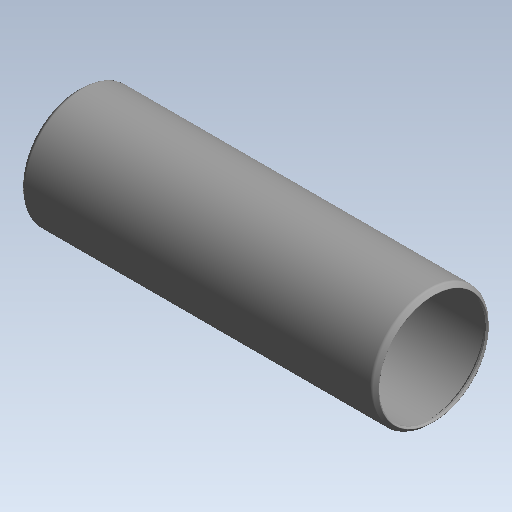
# Autodesk Inventor part: 09R-3.31350SR
Saved by Autodesk Inventor 2020 (Build 240168000, 168)
## iProperties
Part Number: 09R-3.31350SR
Material: Generic
Catalog Web Link: www.cadenas.de
Description: Tube-Original Line - Standard Air Cylinders
Vendor: BIMBA
Document SubType Name: Modeling
Designer: partserver
Manufacturer: BIMBA
Mass: 3.98472 g
Surface Area: 150.377 cm^2
Volume: 3.98472 cm^3
Density: 1 g/cm^3
Appearance: PSOLRGB-180-180-180
Category: PARTsolutions
Company: BIMBA
PSOL_IDENT_0: {$CADENAS_DATA\23d-libs\bimba\bimba_brand\bimba_imperial\bimba_full_line\original_line_cylinders\sta
PSOL_IDENT_1: ndard_air_cylinders\tube.prj},205 {VTYP=3D},{NB=09R-3.31350SR},{LINA=09R-3.31350SR},{NN=Tube},{DATE=
PSOL_IDENT_2: 19.01.2022 10:19:38},{GEOMDATE=03.03.2020 12:52:40},{VERSION=},{LINEID=60},{WBVAR=MNT,ACTING,NR,L,FO
PSOL_IDENT_3: URHOLES,SR,K},{WBNUMERIC=L,FOURHOLES}  {NB=09R-3.31350SR},{LINA=09R-3.31350SR},{KT=DUMMY},{PN=09R-3.
PSOL_IDENT_4: 31350SR},{BORE=1.06250000},{BOREPN=09},{MNT=},{MNTALG='' , 'Front Nose' , 'BF' , 'Front Block' , 'BF
PSOL_IDENT_5: T' , 'Front Trunnion' , 'A' , 'Adjustable Stroke'},{ACTING=R},{ACTINGALG= '' , 'Single Acting' , 'R'
PSOL_IDENT_6: , 'Reverse/Double Acting' },{NR=},{NRALG= '' , 'N/A' },{L=3.3135},{OD=1.1130},{ODN=1.1130},{ODP=1.1
PSOL_IDENT_7: 130},{ODB=1.1410},{ID=1.0715},{DV=0.00000000},{LV=0.00000000},{LV1=0.00000000},{G=0.0300},{FOURHOLES=
PSOL_IDENT_8: 0},{AA=0.3750},{BB=0.0940},{SR=SR},{SRALG= 'C' , 'Carbon Steel Rod' , 'SR' , '303 Stainless Steel Ro
PSOL_IDENT_9: d' , '' , '303 Stainless Steel Rod'},{KALG= '', 'Standard' , 'K' , 'Ports Rotated 90deg' },{K=}
NB: 09R-3.31350SR
NN: Tube
NT: Original Line - Standard Air Cylinders
NBSYN: $PN.
LINA: 09R-3.31350SR
CATALOG: Bimba Products
BORE: 0
BOREPN: 09
MNT: Front Nose
MNTALG: '' , 'Front Nose' , 'BF' , 'Front Block' , 'BFT' , 'Front Trunnion' , 'A' , 'Adjustable Stroke'
ACTING: Reverse/Double Acting
NR: N/A
L: 3.3135
ODN: 1.113
ODP: 1.113
ODB: 1.141
ID: 1.0715
DV: 0
LV: 0
LV1: 0
G: 0.03
FOURHOLES: 0
AA: 0.375
BB: 0.094
SR: 303 Stainless Steel Rod
K: Standard
SUPPLIER: BIMBA
ARTICLENO: 09R-3.31350SR
BOMINFO: 09R-3.31350SR
CREATOR: CADENAS GmbH
Title: 09R-3.31350SR
Author: Cadenas PARTsolutions
Comments: Original Line - Standard Air Cylinders
Autodesk Inventor part; units mm, degrees
sketch "Sketch_1" plane through (0, 0, 0) normal (0, 0, 1) x (1, 0, 0)
  line L0 (84.1629, 0) -> (0, 0)
  arc A0 (-0.6395, 13.2842) -> (-0.6395, 13.1046) centre (-0.5497, 13.1944) ccw
  line L1 (-0.6395, 13.1046) -> (-0.381, 12.846)
  line L2 (-0.381, 12.846) -> (0, 12.846)
  line L3 (0, 12.846) -> (0.762, 13.608)
  line L4 (0.762, 13.608) -> (83.4009, 13.608)
  line L5 (83.4009, 13.608) -> (84.1629, 12.846)
  line L6 (84.1629, 12.846) -> (84.5439, 12.846)
  line L7 (84.5439, 12.846) -> (84.8024, 13.1046)
  arc A1 (84.8024, 13.1046) -> (84.8024, 13.2842) centre (84.7126, 13.1944) ccw
  line L8 (84.8024, 13.2842) -> (84.1747, 13.9119)
  arc A2 (84.1747, 13.9119) -> (83.6359, 14.1351) centre (83.6359, 13.3731) ccw
  line L9 (83.6359, 14.1351) -> (0.5271, 14.1351)
  arc A3 (0.5271, 14.1351) -> (-0.0118, 13.9119) centre (0.527, 13.3731) ccw
  line L10 (-0.0118, 13.9119) -> (-0.6395, 13.2842)
  constraints: 22 end point, 8 point on circle, 4 centre point
revolve "Revolution1" add sketch "Sketch_1" angle 360 about axis through (84.1629, 0, 0) along (1, 0, 0)
ref_plane "cp1_XY" through (42.0815, 0, 14.1351) normal (1, 0, 0) x (0, 0, -1)
ref_plane "cp1_YZ" through (42.0815, 0, 14.1351) normal (0, 0, -1) x (0, 1, 0)
ref_plane "cp1_ZX" through (42.0815, 0, 14.1351) normal (0, 1, 0) x (1, 0, 0)
ref_plane "cp2_XY" through (42.0815, 14.1351, 0) normal (1, 0, 0) x (0, 0, -1)
ref_plane "cp2_YZ" through (42.0815, 14.1351, 0) normal (0, 0, -1) x (0, 1, 0)
ref_plane "cp2_ZX" through (42.0815, 14.1351, 0) normal (0, 1, 0) x (1, 0, 0)
ref_plane "cp3_XY" through (42.0815, 0, -14.1351) normal (1, 0, 0) x (0, 0, -1)
ref_plane "cp3_YZ" through (42.0815, 0, -14.1351) normal (0, 0, -1) x (0, 1, 0)
ref_plane "cp3_ZX" through (42.0815, 0, -14.1351) normal (0, 1, 0) x (1, 0, 0)
ref_plane "cp4_XY" through (42.0815, -14.1351, 0) normal (1, 0, 0) x (0, 0, -1)
ref_plane "cp4_YZ" through (42.0815, -14.1351, 0) normal (0, 0, -1) x (0, 1, 0)
ref_plane "cp4_ZX" through (42.0815, -14.1351, 0) normal (0, 1, 0) x (1, 0, 0)
ref_plane "tube_front_XY" through (0, 0, 0) normal (1, 0, 0) x (0, 0, -1)
ref_plane "tube_front_YZ" through (0, 0, 0) normal (0, 0, -1) x (0, 1, 0)
ref_plane "tube_front_ZX" through (0, 0, 0) normal (0, 1, 0) x (1, 0, 0)
ref_plane "tube_rear_XY" through (84.1629, 0, 0) normal (1, 0, 0) x (0, 0, -1)
ref_plane "tube_rear_YZ" through (84.1629, 0, 0) normal (0, 0, -1) x (0, 1, 0)
ref_plane "tube_rear_ZX" through (84.1629, 0, 0) normal (0, 1, 0) x (1, 0, 0)
body "Solid1"
